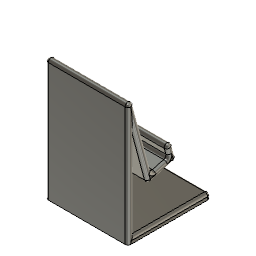
Screen Mount v2 (Autodesk Fusion 360 design; units mm, degrees)
Autodesk Fusion 360 part; units mm, degrees
sketch "Sketch2" plane through (0, 0, 0) normal (1, 0, 0) x (0, 1, 0)
  line L0 (0, 0) -> (70, 0)
  line L1 (0, 0) -> (0, 101.010615)
  line L2 (4.914815, 101.657662) -> (20.058476, 45.140748)
  line L3 (0, 120) -> (80, 120) construction
  line L4 (23.120338, 43.372982) -> (32.779596, 45.961172)
  line L5 (34.547363, 49.023034) -> (32.606221, 56.267478)
  line L6 (5, 5) -> (70, 5)
  line L7 (5, 5) -> (5, 82.021229)
  line L8 (5, 82.021229) -> (16.522942, 39.017024)
  line L9 (19.584804, 37.249257) -> (38.903321, 42.425638)
  line L10 (40.671088, 45.4875) -> (37.43585, 57.561573)
  line L11 (32.606221, 56.267478) -> (37.43585, 57.561573)
  line L12 (70, 0) -> (70, 5)
  arc A0 (37.43585, 57.561573) -> (32.606221, 56.267478) centre (35.021035, 56.914525) ccw
  arc A1 (70, 0) -> (70, 5) centre (70, 2.5) ccw
  arc A2 (4.914815, 101.657662) -> (0, 101.010615) centre (2.5, 101.010615) ccw
  arc A3 (16.522942, 39.017024) -> (19.584804, 37.249257) centre (18.937757, 39.664072) ccw
  arc A4 (38.903321, 42.425638) -> (40.671088, 45.4875) centre (38.256273, 44.840453) ccw
  arc A5 (20.058476, 45.140748) -> (23.120338, 43.372982) centre (22.473291, 45.787796) ccw
  arc A6 (32.779596, 45.961172) -> (34.547363, 49.023034) centre (32.132549, 48.375987) ccw
  point P0 (20.705524, 42.725934)
  point P1 (35.194411, 46.60822)
  dimension "d7" = 70
  dimension "d8" = 120
  dimension "d9" = 80
  dimension "d10" = 75
  dimension "d11" = 15
  dimension "d12" = 10
  dimension "d16" = 2.5
  dimension "d17" = 2.5
  dimension "d18" = 2.5
  dimension "d19" = 2.5
  dimension "d20" = 2.5
  dimension "d21" = 2.5
  dimension "d22" = 2.5
  constraint coincident L0.start L1.start
  constraint horizontal L0
  constraint perpendicular L0 L1
  constraint horizontal L3
  constraint perpendicular L2 L4
  constraint perpendicular L4 L5
  constraint perpendicular L10 L11
  constraint perpendicular L6 L12
  constraint coincident L12.end L6
  constraint coincident L3.start L1
  constraint coincident L3.start L2
  constraint tangent L1 A2
  constraint tangent L2 A2
  constraint tangent L8 A3
  constraint tangent L9 A3
  constraint tangent L9 A4
  constraint tangent L10 A4
  constraint tangent L2 A5
  constraint tangent L4 A5
  constraint tangent L5 A6
  constraint tangent L4 A6
  measures "d7" distance of L0.start L0.end
  measures "d8" distance of L0.start L3.start
  measures "d10" angle of L2 L3
  measures "d16" radius of A0
  measures "d17" radius of A1
  measures "d18" radius of A2
  measures "d19" radius of A3
  measures "d20" radius of A4
  measures "d21" radius of A5
  measures "d22" radius of A6
extrude "Extrude1" add sketch "Sketch2" along normal blind 70 contours L0 L1 L2 L4 L5 L6 L7 L8 L9 L10 L11 L12 A2 A3 A4 A5 A6 picked at (1.666667, 61.010615)
fillet "Fillet1" radius 2.5 1 edges at (35, 37.43585, 57.561573)
fillet "Fillet2" radius 2.5 1 edges at (35, 32.606221, 56.267478)
fillet "Fillet3" radius 2.5 13 edges at (70, 10.761471, 60.519127) (70, 17.687757, 37.499008) (70, 29.244063, 39.837448) (70, 40.421337, 43.590453) (70, 39.376993, 50.317129) (70, 35.021035, 56.914525) (70, 33.900316, 51.437849) (70, 34.297612, 47.125987) (70, 27.949967, 44.667077) (70, 21.223291, 43.622733) (70, 12.486645, 73.399205) (70, 2.173685, 103.489227) (70, 0, 50.505307)
fillet "Fillet4" radius 2.5 1 edges at (70, 5, 48.340244)
fillet "Fillet5" radius 2.5 1 edges at (70, 36.25, 5)
fillet "Fillet6" radius 2.5 3 edges at (33.75, 70, 5) (69.267767, 70, 4.267767) (70, 70, 1.25)
fillet "Fillet7" radius 2.5 13 edges at (0, 0, 50.505307) (0, 2.173685, 103.489227) (0, 12.486645, 73.399205) (0, 21.223291, 43.622733) (0, 27.949967, 44.667077) (0, 34.297612, 47.125987) (0, 33.900316, 51.437849) (0, 35.021035, 56.914525) (0, 39.376993, 50.317129) (0, 40.421337, 43.590453) (0, 29.244063, 39.837448) (0, 17.687757, 37.499008) (0, 10.761471, 60.519127)
fillet "Fillet8" radius 2.5 1 edges at (0, 5, 48.340244)
fillet "Fillet9" radius 2.5 3 edges at (0, 35, 5) (0, 69.267767, 4.267767) (0, 70, 1.25)
